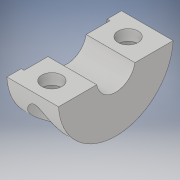
# Autodesk Inventor part: Swivel Joint Axle Lock Side B
Saved by Autodesk Inventor 2019 (Build 230136000, 136)
## iProperties
Created: 2020-04-05
Part Number: Swivel Joint Axle Lock Side B
Material: Generic
Document SubType Name: Modeling
Designer: isaac
Density: 1 g/cm^3
Appearance: Default
Author: isaac
Autodesk Inventor part; units mm, degrees
ref_plane "YZ Plane" through (0, 0, 0) normal (1, 0, 0) x (0, 1, 0)
ref_plane "XY Plane" through (0, 0, 0) normal (0, 0, 1) x (1, 0, 0)
sketch "Sketch1" plane through (0, 0, 0) normal (1, 0, 0) x (0, 1, 0)
  circle A0 centre (0, 0) radius 3.375 construction
  circle A1 centre (0, 0) radius 10 construction
  arc A2 (0.5861, -3.3237) -> (-0.5861, -3.3237) centre (0, 0) ccw
  line L0 (0, 0) -> (0.5861, -3.3237) construction
  line L1 (0, 0) -> (3.375, 0) construction
  line L2 (0, 0) -> (-0.5861, -3.3237) construction
  line L3 (0.5861, -3.3237) -> (0.5861, -9.9828)
  line L4 (-0.5861, -3.3237) -> (-0.5861, -9.9828)
  arc A3 (0.5861, -9.9828) -> (-0.5861, -9.9828) centre (0, 0) ccw
  line L5 (0.5861, -3.3237) -> (0.5861, -9.9828)
  line L6 (-0.5861, -3.3237) -> (-0.5861, -9.9828)
  arc A4 (0.5861, -3.3237) -> (-0.5861, -3.3237) centre (0, 0) ccw
  arc A5 (0.5861, -9.9828) -> (-0.5861, -9.9828) centre (0, 0) ccw
  dimension "d0" = 6.75
  dimension "d1" = 20
  dimension "d2" = 80
  dimension "d3" = 20
  constraints: 14 end point, 11 point on circle, 6 coincident, 5 centre point, 3 equal length, 2 vertical, 1 concentric, 1 horizontal, 3 other
  measures "d1" diameter of A1
  measures "d2" angle of L0 L1
  measures "d3" angle of L2 L0
extrude "Extrusion1" add sketch "Sketch1" against normal blind 9
sketch "Sketch3" plane through (-9, 0, 0) normal (-1, 0, 0) x (0, 0, 1)
  circle A0 centre (0, 0) radius 7.5
  dimension "d9" = 15
  constraints: 1 centre point, 1 coincident
  measures "d9" diameter of A0
extrude "Extrusion3" cut sketch "Sketch3" against normal blind 0.5
ref_plane "Work Plane1" through (0, 10, 0) normal (0, 1, 0) x (-1, 0, 0)
sketch "Sketch4" plane through (0, 10, 0) normal (0, 1, 0) x (-1, 0, 0)
  line L0 (9, 7.5) -> (9, -7.4771) construction
  line L1 (0, -9.9828) -> (9, -9.9828) construction
  line L2 (9, -3.2928) -> (0, -3.2928) construction
  line L3 (0, -3.2928) -> (0, -9.9828) construction
  line L4 (0, -9.9828) -> (9, -9.9828) construction
  line L5 (9, -9.9828) -> (9, -3.2928) construction
  line L6 (9, -3.2928) -> (0, -9.9828) construction
  line L7 (0, -3.2928) -> (9, -9.9828) construction
  line L8 (1.3246, -6.6378) -> (2.9123, -3.8878)
  line L9 (2.9123, -3.8878) -> (6.0877, -3.8878)
  line L10 (6.0877, -3.8878) -> (7.6754, -6.6378)
  line L11 (7.6754, -6.6378) -> (6.0877, -9.3878)
  line L12 (6.0877, -9.3878) -> (2.9123, -9.3878)
  line L13 (2.9123, -9.3878) -> (1.3246, -6.6378)
  point P0 (0, 0)
  point P1 (4.5, -6.6378)
  dimension "d13" = 5.5
  constraints: 24 end point, 2 parallel, 1 horizontal, 1 midpoint, 1 perpendicular, 1 point on line, 13 other
  measures "d13" distance between parallel lines of L12 L9
extrude "Extrusion4" cut sketch "Sketch4" against normal blind 7.5
ref_plane "Work Plane2" through (0, -10, 0) normal (0, 1, 0) x (-1, 0, 0)
sketch "Sketch5" plane through (0, -10, 0) normal (0, 1, 0) x (-1, 0, 0)
  line L0 (2.9123, -9.3878) -> (1.3246, -6.6378) construction
  line L1 (6.0877, -3.8878) -> (7.6754, -6.6378) construction
  line L2 (1.3246, -6.6378) -> (7.6754, -6.6378) construction
  line L3 (2.9123, -3.8878) -> (6.0877, -3.8878) construction
  line L4 (4.5, -3.8878) -> (4.5, -9.3878) construction
  line L5 (6.0877, -9.3878) -> (2.9123, -9.3878) construction
  point P0 (0, 0)
  point P1 (4.5, -6.6378)
  constraints: 4 end point, 3 midpoint, 1 horizontal
hole "Hole1" at (-4.5, -10, -6.6378) direction (0, 1, 0) diameter 3.5 end through all counterbore diameter 6 counterbore depth 7.5
mirror "Mirror1" about plane through (0, 0, 0) normal (0, 0, 1) of "Hole1", "Extrusion4"
sketch "Sketch9" plane through (-9, 0, 0) normal (-1, 0, 0) x (0, 0, 1)
  line L0 (-9.9828, -0.5861) -> (-3.3237, -0.5861) projected
  line L1 (-9.9828, -0.5861) -> (12.5861, -0.5861)
  line L2 (12.5861, -0.5861) -> (12.5861, 15.0406)
  line L3 (12.5861, 15.0406) -> (-9.9828, 15.0406)
  line L4 (-9.9828, 15.0406) -> (-9.9828, -0.5861)
  point P0 (0, 0)
  constraints: 8 end point, 2 parallel, 1 horizontal, 1 perpendicular
extrude "Extrusion6" cut sketch "Sketch9" against normal through all
body "Solid1"
